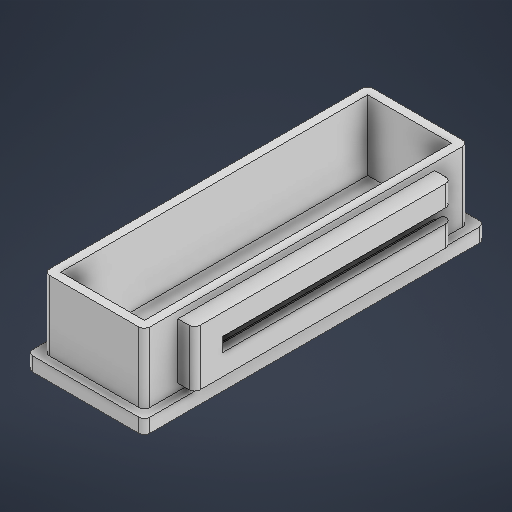
# Autodesk Inventor part: module_switch
Saved by Autodesk Inventor 2025.2 (Build 292293000, 293)
## iProperties
Created: 2025-09-07
Part Number: module_switch
Material: Generic
Document SubType Name: Modeling
Designer: sam
Density: 1 g/cm^3
Appearance: Default
Author: sam
Autodesk Inventor part; units mm, degrees
ref_plane "YZ Plane" through (0, 0, 0) normal (1, 0, 0) x (0, 1, 0)
ref_plane "XZ Plane" through (0, 0, 0) normal (0, 1, 0) x (-1, 0, 0)
ref_plane "XY Plane" through (0, 0, 0) normal (0, 0, 1) x (1, 0, 0)
sketch "Sketch2" plane through (0, 0, 0) normal (0, 1, 0) x (-1, 0, 0)
  line L0 (-21, -61) -> (21, -61)
  line L1 (21, -61) -> (21, 61)
  line L2 (21, 61) -> (-21, 61)
  line L3 (-21, 61) -> (-21, -61)
  line L4 (-21, -61) -> (21, 61) construction
  line L5 (21, -61) -> (-21, 61) construction
  point P0 (0, 0)
  dimension "d0" = 42
  dimension "d1" = 122
  constraints: 12 end point, 2 midpoint, 2 parallel, 1 horizontal, 1 perpendicular
  measures "d0" distance of L2.end L1.end
  measures "d1" distance of L1.end L0.end
extrude "Extrusion1" add sketch "Sketch2" along normal blind 5
sketch "Sketch3" plane through (0, 5, 0) normal (0, 1, 0) x (1, 0, 0)
  line L0 (18, 58) -> (-18, 58)
  line L1 (-18, 58) -> (-18, -58)
  line L2 (-18, -58) -> (18, -58)
  line L3 (18, -58) -> (18, 58)
  line L4 (18, 58) -> (-18, -58) construction
  line L5 (-18, 58) -> (18, -58) construction
  line L6 (-21, 61) -> (-21, -61) projected
  line L7 (-21, -61) -> (21, -61) projected
  line L8 (15, 55) -> (-15, 55)
  line L9 (-15, 55) -> (-15, -55)
  line L10 (-15, -55) -> (15, -55)
  line L11 (15, -55) -> (15, 55)
  line L12 (15, 55) -> (-15, -55) construction
  line L13 (-15, 55) -> (15, -55) construction
  point P0 (0, 0)
  dimension "d4" = 3
  dimension "d5" = 3
  dimension "d6" = 3
  dimension "d7" = 3
  constraints: 24 end point, 4 midpoint, 4 parallel, 2 horizontal, 2 perpendicular
  measures "d4" distance between parallel lines of L6 L1
  measures "d5" distance between parallel lines of L7 L2
  measures "d6" distance between parallel lines of L2 L10
  measures "d7" distance between parallel lines of L1 L9
extrude "Extrusion2" add sketch "Sketch3" along normal blind 25
fillet "Fillet1" radius 2 8 edges at (18, 17.5, 58) (-18, 17.5, 58) (-21, 2.5, 61) (21, 2.5, 61) (18, 17.5, -58) (-18, 17.5, -58) (21, 2.5, -61) (-21, 2.5, -61)
sketch "Sketch4" plane through (18, 5, 56) normal (1, 0, 0) x (0, 0, -1)
  line L0 (10, 22.5) -> (102, 22.5)
  line L1 (102, 22.5) -> (102, 2.5)
  line L2 (102, 2.5) -> (10, 2.5)
  line L3 (10, 2.5) -> (10, 22.5)
  line L4 (112, 25) -> (112, 0) projected
  line L5 (0, 25) -> (112, 25) projected
  line L6 (0, 0) -> (0, 25) projected
  line L7 (112, 0) -> (0, 0) projected
  point P0 (56, -5)
  dimension "d11" = 10
  dimension "d12" = 10
  dimension "d13" = 2.5
  dimension "d14" = 2.5
  constraints: 8 end point, 2 parallel, 1 horizontal, 1 perpendicular
  measures "d11" distance between parallel lines of L3 L6
  measures "d12" distance between parallel lines of L4 L1
  measures "d13" distance between parallel lines of L5 L0
  measures "d14" distance between parallel lines of L7 L2
extrude "Extrusion3" add sketch "Sketch4" along normal blind 6 contours L0 L1 L2 L3
sketch "Sketch5" plane through (18, 7.5, -46) normal (0, 0, -1) x (-1, 0, 0)
  line L0 (0, 20) -> (0, 0) projected
  line L1 (0, 20) -> (-6, 20) projected
  line L2 (-6, 0) -> (-6, 20) projected
  line L3 (0, 0) -> (-6, 0) projected
  line L4 (-6, 12.5) -> (-3, 12.5)
  line L5 (-3, 12.5) -> (-3, 7.5)
  line L6 (-3, 7.5) -> (-6, 7.5)
  line L7 (-6, 7.5) -> (-6, 12.5)
  line L8 (0, 15) -> (-3, 15)
  line L9 (-3, 15) -> (-3, 5)
  line L10 (-3, 5) -> (0, 5)
  line L11 (0, 5) -> (0, 15)
  point P0 (18, -7.5)
  point P1 (-4.5, 7.5)
  point P2 (-4.5, 12.5)
  point P3 (-6, 7.5)
  point P4 (-3, 7.5)
  point P5 (0, 5)
  dimension "d17" = 3
  dimension "d18" = 7.5
  dimension "d19" = 7.5
  dimension "d20" = 5
  dimension "d21" = 5
  constraints: 16 end point, 4 parallel, 3 point on line, 2 horizontal, 2 midpoint, 2 perpendicular
  measures "d17" distance of L5.end L6.end
  measures "d18" distance from line of L3 point (-4.5, 7.5)
  measures "d19" distance from line of point (-4.5, 12.5) L1
  measures "d20" distance between parallel lines of L3 L10
  measures "d21" distance between parallel lines of L1 L8
extrude "Extrusion4" cut sketch "Sketch5" against normal blind 82 contours L0 L10 L9 L5 L8 | L4 L5 L6 L2
sketch "Sketch6" plane through (-18, 5, -56) normal (-1, 0, 0) x (0, 0, 1)
  line L0 (0, 0) -> (0, 25) projected
  line L1 (112, 0) -> (0, 0) projected
  line L2 (112, 25) -> (112, 0) projected
  line L3 (0, 25) -> (112, 25) projected
  line L4 (10, 17.5) -> (92, 17.5)
  line L5 (92, 17.5) -> (92, 7.5)
  line L6 (92, 7.5) -> (10, 7.5)
  line L7 (10, 7.5) -> (10, 17.5)
  point P0 (56, -5)
  dimension "d24" = 10
  dimension "d25" = 20
  dimension "d26" = 7.5
  dimension "d27" = 7.5
  constraints: 8 end point, 2 parallel, 1 horizontal, 1 perpendicular
  measures "d24" distance between parallel lines of L0 L7
  measures "d25" distance between parallel lines of L2 L5
  measures "d26" distance between parallel lines of L3 L4
  measures "d27" distance between parallel lines of L1 L6
extrude "Extrusion5" add sketch "Sketch6" along normal blind 6 contours L4 L5 L6 L7
sketch "Sketch7" plane through (-18, 12.5, 36) normal (0, 0, 1) x (1, 0, 0)
  line L0 (0, 10) -> (0, 0) projected
  line L1 (0, 10) -> (-6, 10) projected
  line L2 (-6, 0) -> (-6, 10) projected
  line L3 (0, 0) -> (-6, 0) projected
  line L4 (0, 10) -> (-3, 10)
  line L5 (-3, 10) -> (-3, 7.5)
  line L6 (-3, 7.5) -> (0, 7.5)
  line L7 (0, 7.5) -> (0, 10)
  line L8 (0, 0) -> (-3, 0)
  line L9 (-3, 0) -> (-3, 2.5)
  line L10 (-3, 2.5) -> (0, 2.5)
  line L11 (0, 2.5) -> (0, 0)
  point P0 (18, -12.5)
  dimension "d30" = 3
  dimension "d31" = 2.5
  dimension "d32" = 3
  dimension "d33" = 2.5
  constraints: 16 end point, 4 parallel, 2 horizontal, 2 perpendicular
  measures "d30" distance of L6.end L5.end
  measures "d31" distance of L5.end L4.end
  measures "d32" distance of L9.end L10.end
  measures "d33" distance of L8.end L9.end
extrude "Extrusion6" cut sketch "Sketch7" against normal through all contours L0 L6 L5 L1 | L0 L3 L9 L10
fillet "Fillet3" radius 1 4 edges at (-19.5, 20, -46) (-19.5, 15, -46) (-19.5, 20, 36) (-19.5, 15, 36)
fillet "Fillet4" radius 1 4 edges at (-24, 22.5, -5) (-21, 22.5, -5) (-24, 12.5, -5) (-21, 12.5, -5)
fillet "Fillet5" radius 2 3 edges at (24, 17.5, 46) (24, 23.75, -46) (24, 11.25, -46)
fillet "Fillet6" radius 1 11 edges at (-23.7071, 22.2071, 36) (-22.5, 22.5, 36) (-21.2929, 22.2071, 36) (-21, 19.5, 36) (-21, 20.75, 36) (-23.7071, 12.7929, 36) (-22.5, 12.5, 36) (-21.2929, 12.7929, 36) (-21, 14.25, 36) (-21, 15.5, 36) (-24, 17.5, 36)
fillet "Fillet7" radius 1 11 edges at (-21.2929, 22.2071, -46) (-22.5, 22.5, -46) (-23.7071, 22.2071, -46) (-24, 17.5, -46) (-23.7071, 12.7929, -46) (-22.5, 12.5, -46) (-21.2929, 12.7929, -46) (-21, 15.5, -46) (-21, 14.25, -46) (-21, 20.75, -46) (-21, 19.5, -46)
body "Solid1"
